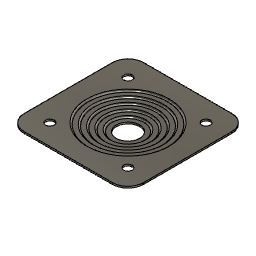
TapaBaseReloj V2 (Autodesk Fusion 360 design; units mm, degrees)
Autodesk Fusion 360 part; units mm, degrees
sketch "Boceto1" plane through (0, 0, 0) normal (0, 0, 1) x (1, 0, 0)
  line L0 (77, -77) -> (-77, -77)
  line L1 (-77, -77) -> (-77, 77)
  line L2 (-77, 77) -> (77, 77)
  line L3 (77, 77) -> (77, -77)
  line L4 (77, -77) -> (-77, 77) construction
  line L5 (-77, -77) -> (77, 77) construction
  dimension "d1" = 154
  dimension "d2" = 154
  constraint horizontal L0
  constraint perpendicular L0 L1
  constraint parallel L0 L2
  constraint parallel L1 L3
  constraint coincident L4 origin
  constraint coincident L5 origin
  measures "d1" distance of L1.end L2.end
  measures "d2" distance of L0.end L1.end
extrude "Extruir1" add sketch "Boceto1" along normal blind 2
fillet "Empalme1" radius 20 4 edges at (-77, -77, 1) (77, -77, 1) (-77, 77, 1) (77, 77, 1)
sketch "Boceto2" plane through (0, 0, 2) normal (0, 0, 1) x (-1, 0, 0)
  arc A0 (-77, -57) -> (-57, -77) centre (-57, -57) ccw
  line L0 (-57, -77) -> (57, -77)
  arc A1 (57, -77) -> (77, -57) centre (57, -57) ccw
  line L1 (77, -57) -> (77, 57)
  arc A2 (77, 57) -> (57, 77) centre (57, 57) ccw
  line L2 (57, 77) -> (-57, 77)
  arc A3 (-57, 77) -> (-77, 57) centre (-57, 57) ccw
  line L3 (-77, 57) -> (-77, -57)
  circle A4 centre (50, -50) radius 5.5
  circle A5 centre (-50, -50) radius 5.5
  circle A6 centre (-50, 50) radius 5.5
  circle A7 centre (50, 50) radius 5.5
  dimension "d7" = 11
  dimension "d8" = 11
  dimension "d9" = 11
  dimension "d10" = 11
  measures "d7" diameter of A4
  measures "d8" diameter of A5
  measures "d9" diameter of A6
  measures "d10" diameter of A7
extrude "Extruir2" cut sketch "Boceto2" against normal blind 21 contours A4 | A5 | A6 | A7
sketch "Boceto3" plane through (0, 0, 2) normal (0, 0, 1) x (-1, 0, 0)
  circle A0 centre (50, 50) radius 5.5
  circle A1 centre (-50, -50) radius 5.5
  circle A2 centre (-50, 50) radius 5.5
  circle A3 centre (50, -50) radius 5.5
  arc A4 (-77, -57) -> (-57, -77) centre (-57, -57) ccw
  line L0 (-57, -77) -> (57, -77)
  arc A5 (57, -77) -> (77, -57) centre (57, -57) ccw
  line L1 (77, -57) -> (77, 57)
  arc A6 (77, 57) -> (57, 77) centre (57, 57) ccw
  line L2 (57, 77) -> (-57, 77)
  arc A7 (-57, 77) -> (-77, 57) centre (-57, 57) ccw
  line L3 (-77, 57) -> (-77, -57)
  circle A8 centre (0, 0) radius 52.5
  dimension "d13" = 105
  constraint coincident A8.centre origin
  measures "d13" diameter of A8
extrude "Extruir3" cut sketch "Boceto3" against normal blind 2 contours A8
sketch "Boceto4" plane through (0, 0, 0) normal (0, 0, -1) x (1, 0, 0)
  circle A0 centre (0, 0) radius 52.5
  circle A1 centre (-50, 50) radius 5.5
  circle A2 centre (50, -50) radius 5.5
  circle A3 centre (50, 50) radius 5.5
  circle A4 centre (-50, -50) radius 5.5
  arc A5 (57, -77) -> (77, -57) centre (57, -57) ccw
  line L0 (77, -57) -> (77, 57)
  arc A6 (77, 57) -> (57, 77) centre (57, 57) ccw
  line L1 (57, 77) -> (-57, 77)
  arc A7 (-57, 77) -> (-77, 57) centre (-57, 57) ccw
  line L2 (-77, 57) -> (-77, -57)
  arc A8 (-77, -57) -> (-57, -77) centre (-57, -57) ccw
  line L3 (-57, -77) -> (57, -77)
  circle A9 centre (0, 0) radius 60
  dimension "d16" = 120
  constraint concentric A0 A9
  measures "d16" diameter of A9
extrude "Extruir4" add sketch "Boceto4" along normal blind 2 contours A0 | A9
sketch "Boceto5" plane through (0, 0, 0) normal (0, 0, 1) x (-1, 0, 0)
  circle A0 centre (0, 0) radius 52.5
  circle A1 centre (0, 0) radius 45
  constraint coincident A0.centre A1.centre
extrude "Extruir5" cut sketch "Boceto5" against normal blind 20 contours A1
sketch "Boceto6" plane through (0, 0, -2) normal (0, 0, -1) x (1, 0, 0)
  circle A0 centre (0, 0) radius 45
  circle A1 centre (0, 0) radius 60
  circle A2 centre (0, 0) radius 52.5
  dimension "d21" = 105
  constraint coincident A0.centre A1.centre
  measures "d21" diameter of A2
extrude "Extruir6" add sketch "Boceto6" along normal blind 2 contours A0 | A2
sketch "Boceto7" plane through (0, 0, -2) normal (0, 0, 1) x (-1, 0, 0)
  circle A0 centre (0, 0) radius 45
  circle A1 centre (0, 0) radius 37.5
  dimension "d24" = 75
  constraint coincident A0.centre A1.centre
  measures "d24" diameter of A1
extrude "Extruir7" cut sketch "Boceto7" against normal blind 20 contours A1
sketch "Boceto8" plane through (0, 0, -4) normal (0, 0, -1) x (1, 0, 0)
  circle A0 centre (0, 0) radius 37.5
  circle A1 centre (0, 0) radius 52.5
  circle A2 centre (0, 0) radius 45
  dimension "d27" = 90
  constraint concentric A0 A2
  measures "d27" diameter of A2
extrude "Extruir8" add sketch "Boceto8" along normal blind 2 contours A0 | A2
sketch "Boceto9" plane through (0, 0, -4) normal (0, 0, 1) x (-1, 0, 0)
  circle A0 centre (0, 0) radius 37.5
  circle A1 centre (0, 0) radius 30
  dimension "d30" = 60
  constraint concentric A0 A1
  measures "d30" diameter of A1
extrude "Extruir9" cut sketch "Boceto9" against normal blind 2 contours A1
sketch "Boceto10" plane through (0, 0, -6) normal (0, 0, -1) x (1, 0, 0)
  circle A0 centre (0, 0) radius 30
  circle A1 centre (0, 0) radius 45
  circle A2 centre (0, 0) radius 37.5
  dimension "d33" = 75
  constraint coincident A0.centre A1.centre
  measures "d33" diameter of A2
extrude "Extruir10" add sketch "Boceto10" along normal blind 2 contours A0 | A2
sketch "Boceto11" plane through (0, 0, -6) normal (0, 0, 1) x (-1, 0, 0)
  circle A0 centre (0, 0) radius 30
  circle A1 centre (0, 0) radius 22.5
  dimension "d36" = 45
  constraint concentric A0 A1
  measures "d36" diameter of A1
extrude "Extruir11" cut sketch "Boceto11" against normal blind 2 contours A1
sketch "Boceto12" plane through (0, 0, -8) normal (0, 0, -1) x (1, 0, 0)
  circle A0 centre (0, 0) radius 22.5
  circle A1 centre (0, 0) radius 37.5
  circle A2 centre (0, 0) radius 30
  constraint concentric A0 A2
extrude "Extruir12" add sketch "Boceto12" along normal blind 2 contours A0 | A2
sketch "Boceto13" plane through (0, 0, -8) normal (0, 0, 1) x (-1, 0, 0)
  circle A0 centre (0, 0) radius 22.5
  circle A1 centre (0, 0) radius 15
  dimension "d41" = 30
  constraint coincident A0.centre A1.centre
  measures "d41" diameter of A1
extrude "Extruir13" cut sketch "Boceto13" against normal blind 2 contours A1
fillet "Empalme2" radius 2 1 edges at (48.9472, 18.9848, 0)
fillet "Empalme3" radius 2 4 edges at (41.9547, 16.2727, -2) (34.9623, 13.5606, -4) (27.9698, 10.8485, -6) (20.9774, 8.1363, -8)
sketch "Boceto14" plane through (0, 0, 2) normal (0, 0, 1) x (-1, 0, 0)
  circle A0 centre (0, 0) radius 52.5
  circle A1 centre (50, 50) radius 5.5
  circle A2 centre (-50, -50) radius 5.5
  circle A3 centre (-50, 50) radius 5.5
  circle A4 centre (50, -50) radius 5.5
  arc A5 (-77, -57) -> (-57, -77) centre (-57, -57) ccw
  line L0 (-57, -77) -> (57, -77)
  arc A6 (57, -77) -> (77, -57) centre (57, -57) ccw
  line L1 (77, -57) -> (77, 57)
  arc A7 (77, 57) -> (57, 77) centre (57, 57) ccw
  line L2 (57, 77) -> (-57, 77)
  arc A8 (-57, 77) -> (-77, 57) centre (-57, 57) ccw
  line L3 (-77, 57) -> (-77, -57)
  line L4 (76.5, -76.5) -> (-76.5, -76.5)
  line L5 (-76.5, -76.5) -> (-76.5, 76.5)
  line L6 (-76.5, 76.5) -> (76.5, 76.5)
  line L7 (76.5, 76.5) -> (76.5, -76.5)
  line L8 (76.5, -76.5) -> (-76.5, 76.5) construction
  line L9 (-76.5, -76.5) -> (76.5, 76.5) construction
  line L10 (77, -77) -> (-77, -77)
  line L11 (-77, -77) -> (-77, 77)
  line L12 (-77, 77) -> (77, 77)
  line L13 (77, 77) -> (77, -77)
  line L14 (77, -77) -> (-77, 77) construction
  line L15 (-77, -77) -> (77, 77) construction
  arc A9 (57, -77) -> (77, -57) centre (57, -57) ccw
  dimension "d48" = 153
  dimension "d49" = 153
  dimension "d50" = 154
  dimension "d51" = 154
  constraint horizontal L4
  constraint perpendicular L4 L5
  constraint parallel L4 L6
  constraint parallel L5 L7
  constraint coincident L8 A0.centre
  constraint coincident L9 A0.centre
  constraint coincident A0.centre origin
  constraint horizontal L10
  constraint perpendicular L10 L11
  constraint parallel L10 L12
  constraint parallel L11 L13
  constraint coincident L14 A0.centre
  constraint coincident L15 A0.centre
  constraint coincident A6.end L1.start
  constraint coincident L0.end A6.start
  measures "d48" distance of L5.end L6.end
  measures "d49" distance of L4.end L5.end
  measures "d50" distance of L11.end L12.end
  measures "d51" distance of L10.end L11.end
extrude "Extruir14" cut sketch "Boceto14" against normal blind 3 contours A5 A8 L3 L5 L11 | A5 L0 A6 L4 L10 A9 | A7 L2 A8 L6 L12 | A6 L1 A7 L7 L13 A9
sketch "Boceto15" plane through (0, 0, 2) normal (0, 0, 1) x (-1, 0, 0)
  circle A0 centre (50, -50) radius 5.5
  circle A1 centre (-50, 50) radius 5.5
  circle A2 centre (-50, -50) radius 5.5
  circle A3 centre (50, 50) radius 5.5
  circle A4 centre (0, 0) radius 52.5
  line L0 (-76.5, 61.4441) -> (-76.5, -61.4441)
  arc A5 (-76.5, -61.4441) -> (-61.4441, -76.5) centre (-57, -57) ccw
  line L1 (-61.4441, -76.5) -> (61.4441, -76.5)
  arc A6 (61.4441, -76.5) -> (76.5, -61.4441) centre (57, -57) ccw
  line L2 (76.5, -61.4441) -> (76.5, 61.4441)
  arc A7 (76.5, 61.4441) -> (61.4441, 76.5) centre (57, 57) ccw
  line L3 (61.4441, 76.5) -> (-61.4441, 76.5)
  arc A8 (-61.4441, 76.5) -> (-76.5, 61.4441) centre (-57, 57) ccw
  line L4 (76.5, -76.5) -> (-76.5, -76.5)
  line L5 (-76.5, -76.5) -> (-76.5, 76.5)
  line L6 (-76.5, 76.5) -> (76.5, 76.5)
  line L7 (76.5, 76.5) -> (76.5, -76.5)
  line L8 (76.5, -76.5) -> (-76.5, 76.5) construction
  line L9 (-76.5, -76.5) -> (76.5, 76.5) construction
  circle A9 centre (57, -57) radius 20
  circle A10 centre (-57, -57) radius 20
  circle A11 centre (-57, 57) radius 20
  circle A12 centre (57, 57) radius 20
  dimension "d54" = 153
  dimension "d55" = 153
  dimension "d56" = 40
  dimension "d57" = 40
  dimension "d58" = 40
  dimension "d59" = 40
  constraint horizontal L4
  constraint perpendicular L4 L5
  constraint parallel L4 L6
  constraint parallel L5 L7
  constraint coincident L8 A4.centre
  constraint coincident L9 A4.centre
  constraint coincident A4.centre origin
  constraint concentric A6 A9
  constraint concentric A5 A10
  constraint concentric A8 A11
  constraint concentric A7 A12
  measures "d54" distance of L5.end L6.end
  measures "d55" distance of L4.end L5.end
  measures "d56" diameter of A9
  measures "d57" diameter of A10
  measures "d58" diameter of A11
  measures "d59" diameter of A12
extrude "Extruir15" add sketch "Boceto15" against normal blind 2 contours A8 L5 L6 A11 | A5 L4 L5 A10 | A7 L6 L7 A12 | A6 L4 L7 A9
fillet "Empalme4" radius 20 4 edges at (-76.5, -76.5, 1) (76.5, -76.5, 1) (76.5, 76.5, 1) (-76.5, 76.5, 1)
